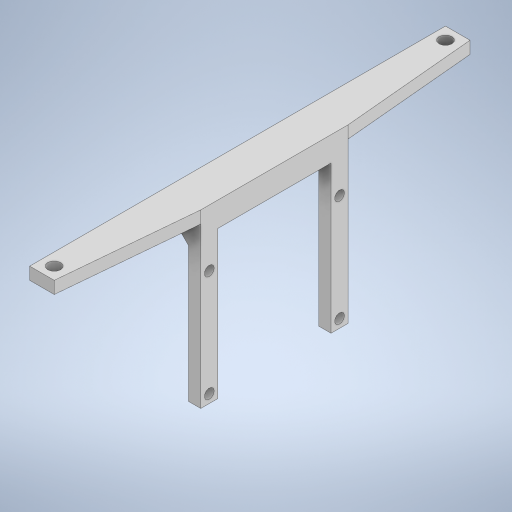
# Autodesk Inventor part: grumpy camera mount
Saved by Autodesk Inventor 2023 (Build 270158000, 158)
## iProperties
Created: 2022-09-13
Part Number: grumpy camera mount
Material: Generic
Document SubType Name: Modeling
Designer: Eli
Density: 1 g/cm^3
Appearance: Default
Author: Eli
Autodesk Inventor part; units mm, degrees
ref_plane "YZ Plane" through (0, 0, 0) normal (1, 0, 0) x (0, 1, 0)
ref_plane "XZ Plane" through (0, 0, 0) normal (0, 1, 0) x (-1, 0, 0)
ref_plane "XY Plane" through (0, 0, 0) normal (0, 0, 1) x (1, 0, 0)
sketch "Sketch1" plane through (0, 0, 0) normal (0, 1, 0) x (-1, 0, 0)
  circle A0 centre (0, 0) radius 1.651
  circle A1 centre (0, -101.1428) radius 1.651
  line L0 (0, 0) -> (0, -101.1428) construction
  line L1 (3.175, 3.175) -> (-6.35, 3.175)
  line L2 (-6.35, 3.175) -> (-6.35, -104.3178)
  line L3 (-6.35, -104.3178) -> (3.175, -104.3178)
  line L4 (3.175, -104.3178) -> (3.175, 3.175)
  dimension "d0" = 3.302
  dimension "d1" = 101.1428
  dimension "d3" = 3.175
  dimension "d4" = 3.175
  dimension "d5" = 3.175
  dimension "d6" = 6.35
  constraints: 10 end point, 2 centre point, 2 parallel, 1 coincident, 1 equal radius, 1 horizontal, 1 perpendicular, 1 vertical
  measures "d0" diameter of A0
  measures "d1" distance of L0.end point (0, 0)
  measures "d3" distance from line of L3 L0.end
  measures "d4" distance from line of point (0, 0) L1
  measures "d5" distance between parallel lines of L4 L0
  measures "d6" distance between parallel lines of L2 L0
extrude "Extrusion1" add sketch "Sketch1" along normal blind 3.175
sketch "Sketch2" plane through (0, 0, 0) normal (0, -1, 0) x (1, 0, 0)
  line L0 (6.35, 3.175) -> (6.35, -104.3178) projected
  line L1 (6.35, -31.5214) -> (3.175, -31.5214)
  line L2 (3.175, -31.5214) -> (3.175, -69.6214)
  line L3 (3.175, -69.6214) -> (6.35, -69.6214)
  line L4 (6.35, -69.6214) -> (6.35, -31.5214)
  line L5 (-3.175, -104.3178) -> (-3.175, 3.175) construction
  line L6 (-3.175, -50.5714) -> (6.35, -50.5714) construction
  point P0 (0, 0)
  dimension "d9" = 38.1
  dimension "d10" = 3.175
  constraints: 10 end point, 2 horizontal, 2 midpoint, 2 parallel, 1 perpendicular, 1 point on line, 1 other
  measures "d9" distance of L1.end L2.end
  measures "d10" distance of L2.end L3.end
extrude "Extrusion2" add sketch "Sketch2" along normal blind 41.275
sketch "Sketch3" plane through (6.35, 0, -104.3178) normal (1, 0, 0) x (0, 0, -1)
  circle A0 centre (-70.5866, -39.0652) radius 1.27
  circle A1 centre (-70.5866, -11.5697) radius 1.27
  circle A2 centre (-36.9062, -11.5697) radius 1.27
  circle A3 centre (-36.9062, -39.0652) radius 1.27
  line L0 (-70.5866, -11.5697) -> (-70.5866, -39.0652) construction
  line L1 (-70.5866, -39.0652) -> (-36.9062, -39.0652) construction
  line L2 (-36.9062, -39.0652) -> (-36.9062, -11.5697) construction
  line L3 (-36.9062, -11.5697) -> (-70.5866, -11.5697) construction
  line L4 (-34.6964, -41.275) -> (-72.7964, -41.275) construction
  line L5 (-53.7464, -41.275) -> (-53.7464, 0) construction
  line L6 (-34.6964, 0) -> (-72.7964, 0) construction
  line L7 (-68.3768, -41.275) -> (-39.116, -41.275)
  line L8 (-39.116, -41.275) -> (-39.116, -3.175)
  line L9 (-39.116, -3.175) -> (-68.3768, -3.175)
  line L10 (-68.3768, -3.175) -> (-68.3768, -41.275)
  line L11 (-72.7964, 0) -> (-72.7964, -41.275) projected
  point P0 (-104.3178, 0)
  dimension "d13" = 2.54
  dimension "d14" = 27.4955
  dimension "d15" = 33.6804
  dimension "d17" = 2.2098
  dimension "d18" = 2.2098
  dimension "d19" = 2.2098
  dimension "d20" = 2.2098
  dimension "d21" = 3.175
  constraints: 18 end point, 4 centre point, 3 equal radius, 3 parallel, 3 perpendicular, 2 midpoint, 1 horizontal, 1 point on line, 1 vertical, 1 other
  measures "d13" diameter of A0
  measures "d14" distance of L0.end L0.start
  measures "d15" distance of L2.end L0.start
  measures "d17" distance between parallel lines of L4 L1
  measures "d18" distance between parallel lines of L0 L10
  measures "d19" distance between parallel lines of L0 L11
  measures "d20" distance between parallel lines of L2 L8
  measures "d21" distance between parallel lines of L6 L9
extrude "Extrusion3" cut sketch "Sketch3" against normal up to surface (3.175 mm away)
chamfer "Chamfer1" distance 6.35 angle 45 1 edges at (3.175, 0, -50.5714)
chamfer "Chamfer2" distance 3.175 distance2 34.6964 1 edges at (6.35, 1.5875, 3.175) measured on face at (0, 1.0583, 3.175)
chamfer "Chamfer3" distance 34.6964 distance2 3.175 1 edges at (6.35, 1.5875, -104.3178) measured on face at (6.35, 2.1167, -68.4869)
body "Solid1"
